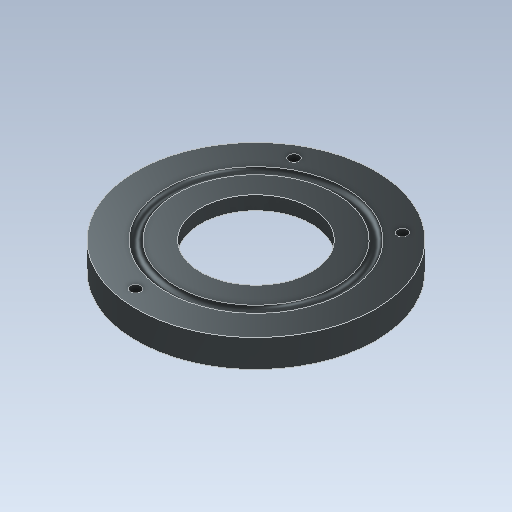
# Autodesk Inventor part: Корпус дросселя_CPY
Saved by Autodesk Inventor 2021 (Build 250183000, 183)
## iProperties
Created: 2020-11-05
Part Number: Корпус дросселя_CPY
Material: Чугун, серый
Document SubType Name: Modeling
Designer: Тимоха
Mass: 1127.79 g
Surface Area: 355.126 cm^2
Volume: 157.733 cm^3
Density: 7.15 g/cm^3
Appearance: Чугун серый
Author: Тимоха
Autodesk Inventor part; units mm, degrees
ref_plane "YZ Plane" through (0, 0, 0) normal (1, 0, 0) x (0, 1, 0)
ref_plane "XZ Plane" through (0, 0, 0) normal (0, 1, 0) x (-1, 0, 0)
ref_plane "XY Plane" through (0, 0, 0) normal (0, 0, 1) x (1, 0, 0)
sketch "Эскиз1" plane through (0, 0, 0) normal (0, 0, 1) x (1, 0, 0)
  line L0 (0, 0) -> (0, 8)
  line L1 (0, 8) -> (0, 16)
  line L2 (0, 16) -> (69, 16)
  line L3 (69, 16) -> (69, 0)
  line L4 (69, 0) -> (49, 0)
  line L5 (49, 0) -> (49, 8)
  line L6 (49, 8) -> (32, 8)
  line L7 (32, 8) -> (32, 16)
  line L8 (0, 16) -> (49, 16)
  line L9 (49, 16) -> (49, 17)
  circle A0 centre (49, 17) radius 3
  point P0 (51.8284, 16)
  point P1 (46.1716, 16)
  dimension "d0" = 8
  dimension "d1" = 8
  dimension "d2" = 69
  dimension "d3" = 20
  dimension "d4" = 17
  dimension "d6" = 32
  dimension "d7" = 49
  dimension "d8" = 49
  dimension "d9" = 1
  dimension "d10" = 6
  constraints: 20 end point, 5 perpendicular, 4 vertical, 2 point on line, 1 centre point, 1 coincident
  measures "d0" distance of L0.start L0.end
  measures "d1" distance of L0.end L1.end
  measures "d2" distance of L1.end L2.end
  measures "d3" distance of L3.end L4.end
  measures "d4" distance of L5.end L6.end
  measures "d6" distance between parallel lines of L0 L7
  measures "d7" distance between parallel lines of L0 L5
  measures "d8" distance of L1.end L8.end
  measures "d9" distance of L8.end L9.end
  measures "d10" diameter of A0
revolve "Вращение1" add sketch "Эскиз1" angle 360 about axis through (0, 8, 0) along (0, 1, 0) contours L2 A0 L3 L4 L5 L6 L7
sketch "Эскиз2" plane through (0, 16, 0) normal (0, 1, 0) x (1, 0, 0)
  line L0 (0, 0) -> (38.5673, 45.9627)
  line L1 (0, 0) -> (60, 0) construction
  line L2 (0, 0) -> (-30, 51.9615)
  line L3 (0, 0) -> (60, 0) construction
  line L4 (0, 0) -> (-10.4189, -59.0885)
  line L5 (0, 0) -> (60, 0) construction
  circle A0 centre (-30, 51.9615) radius 3
  circle A1 centre (38.5673, 45.9627) radius 3
  circle A2 centre (-10.4189, -59.0885) radius 3
  dimension "d11" = 60
  dimension "d12" = 50
  dimension "d13" = 60
  dimension "d14" = 120
  dimension "d15" = 60
  dimension "d16" = 100
  dimension "d17" = 6
  dimension "d18" = 6
  dimension "d19" = 6
  constraints: 12 end point, 3 centre point, 3 coincident, 3 equal length, 3 horizontal
  measures "d11" distance of L0.start L0.end
  measures "d12" angle of L1 L0
  measures "d13" distance of L0.start L2.end
  measures "d14" angle of L3 L2
  measures "d15" distance of L0.start L4.end
  measures "d16" angle of L4 L5
  measures "d17" diameter of A0
  measures "d18" diameter of A1
  measures "d19" diameter of A2
extrude "Выдавливание1" cut sketch "Эскиз2" against normal through all
